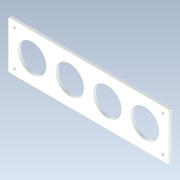
# Autodesk Inventor part: TopPlates
Saved by Autodesk Inventor 2022.2 (Build 262287000, 287)
## iProperties
Created: 2021-12-01
Part Number: TopPlates
Material: Generic
Document SubType Name: Modeling
Designer: Fabijan_Sven
Density: 1 g/cm^3
Appearance: Default
Author: Fabijan_Sven
Autodesk Inventor part; units mm, degrees
ref_plane "YZ Plane" through (0, 0, 0) normal (1, 0, 0) x (0, 1, 0)
ref_plane "XZ Plane" through (0, 0, 0) normal (0, 1, 0) x (-1, 0, 0)
ref_plane "XY Plane" through (0, 0, 0) normal (0, 0, 1) x (1, 0, 0)
sketch "Sketch1" plane through (0, 0, 0) normal (0, 0, 1) x (1, 0, 0)
  line L0 (0, 0) -> (270, 0)
  line L1 (270, 0) -> (270, 80)
  line L2 (270, 80) -> (0, 80)
  line L3 (0, 80) -> (0, 0)
  circle A0 centre (40, 40) radius 24
  circle A1 centre (103.3333, 40) radius 24
  circle A2 centre (166.6667, 40) radius 24
  circle A3 centre (230, 40) radius 24
  dimension "d0" = 270
  dimension "d1" = 80
  dimension "d2" = 40
  dimension "d3" = 63.3333
  dimension "d4" = 63.3333
  dimension "d5" = 63.3333
  dimension "d6" = 48
  dimension "d7" = 48
  dimension "d8" = 48
  dimension "d9" = 48
  constraints: 8 end point, 4 centre point, 2 parallel, 1 horizontal, 1 perpendicular
  measures "d0" distance of L1.end L2.end
  measures "d1" distance of L0.end L1.end
  measures "d2" distance from line of L3 A0.centre
  measures "d3" distance of A1.centre A0.centre
  measures "d4" distance of A1.centre A2.centre
  measures "d5" distance of A2.centre A3.centre
  measures "d6" diameter of A0
  measures "d7" diameter of A1
  measures "d8" diameter of A2
  measures "d9" diameter of A3
extrude "Extrusion1" add sketch "Sketch1" along normal blind 5
sketch "Sketch2" plane through (0, 0, 5) normal (0, 0, 1) x (1, 0, 0)
  circle A0 centre (10, 70) radius 2.75
  circle A1 centre (260, 70) radius 2.75
  circle A2 centre (260, 10) radius 2.75
  circle A3 centre (10, 10) radius 2.75
  line L0 (270, 80) -> (0, 80) projected
  line L1 (0, 80) -> (0, 0) projected
  line L2 (0, 0) -> (270, 0) projected
  line L3 (270, 0) -> (270, 80) projected
  dimension "d12" = 10
  dimension "d13" = 10
  dimension "d14" = 10
  dimension "d15" = 10
  dimension "d16" = 10
  dimension "d17" = 10
  dimension "d18" = 10
  dimension "d19" = 10
  dimension "d20" = 5.5
  dimension "d21" = 5.5
  dimension "d22" = 5.5
  dimension "d23" = 5.5
  constraints: 4 centre point
  measures "d12" distance from line of L0 A0.centre
  measures "d13" distance from line of L1 A0.centre
  measures "d14" distance from line of L1 A3.centre
  measures "d15" distance from line of L2 A3.centre
  measures "d16" distance from line of L0 A1.centre
  measures "d17" distance from line of L3 A1.centre
  measures "d18" distance from line of L3 A2.centre
  measures "d19" distance from line of L2 A2.centre
  measures "d20" diameter of A0
  measures "d21" diameter of A3
  measures "d22" diameter of A1
  measures "d23" diameter of A2
hole "Hole1" at (10, 70, 5) at (260, 70, 5) at (260, 10, 5) at (10, 10, 5) direction (0, 0, -1) diameter 5.5 end through all
fillet "Fillet1" radius 2 4 edges at (0, 0, 2.5) (270, 0, 2.5) (270, 80, 2.5) (0, 80, 2.5)
equation "\"d4\" = d3"
equation "\"d5\" = d3"
equation "\"d7\" = d6"
equation "\"d8\" = d6"
equation "\"d9\" = d6"
equation "\"d13\" = d12"
equation "\"d14\" = d12"
equation "\"d15\" = d12"
equation "\"d16\" = d12"
equation "\"d17\" = d12"
equation "\"d18\" = d12"
equation "\"d19\" = d12"
equation "\"d21\" = d20"
equation "\"d22\" = d20"
equation "\"d23\" = d20"
equation "\"d24\" = d20"
body "Solid1"
